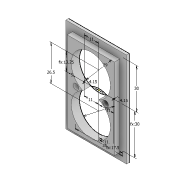
# Autodesk Inventor part: sf11c_lidar_mount
Saved by Autodesk Inventor 2022 (Build 260153000, 153)
## iProperties
Created: 2022-05-19
Part Number: sf11c_lidar_mount
Material: Generic
Document SubType Name: Modeling
Designer: Thomas
Density: 1 g/cm^3
Appearance: Default
Author: Thomas
Autodesk Inventor part; units mm, degrees
ref_plane "YZ Plane" through (0, 0, 0) normal (1, 0, 0) x (0, 1, 0)
ref_plane "XZ Plane" through (0, 0, 0) normal (0, 1, 0) x (-1, 0, 0)
ref_plane "XY Plane" through (0, 0, 0) normal (0, 0, 1) x (1, 0, 0)
sketch "Sketch1" plane through (0, 0, 0) normal (0, 0, 1) x (1, 0, 0)
  circle A0 centre (0, 13.25) radius 14.5
  circle A1 centre (0, -13.25) radius 14.5
  line L0 (0, 13.25) -> (0, -13.25) construction
  circle A2 centre (11, 0) radius 2.075
  circle A3 centre (-11, 0) radius 2.075
  line L1 (-17.5, 30) -> (17.5, 30)
  line L2 (17.5, 30) -> (17.5, -30)
  line L3 (17.5, -30) -> (-17.5, -30)
  line L4 (-17.5, -30) -> (-17.5, 30)
  line L5 (-22.5, 35) -> (22.5, 35)
  line L6 (22.5, 35) -> (22.5, -35)
  line L7 (22.5, -35) -> (-22.5, -35)
  line L8 (-22.5, -35) -> (-22.5, 35)
  point P0 (0, 0)
  point P1 (-5.8896, 0)
  point P2 (5.8896, 0)
  dimension "d0" = 29
  dimension "d1" = 29
  dimension "d2" = 26.5
  dimension "d3" = 13.25
  dimension "d6" = 0
  dimension "d7" = 4.15
  dimension "d8" = 4.15
  dimension "d9" = 11
  dimension "d10" = 11
  dimension "d11" = 11
  dimension "d12" = 11
  dimension "d13" = 35
  dimension "d14" = 17.5
  dimension "d15" = 30
  dimension "d16" = 30
  dimension "d17" = 5
  constraints: 18 end point, 4 centre point, 4 parallel, 2 perpendicular, 1 horizontal, 1 vertical, 3 other
  measures "d0" diameter of A0
  measures "d1" diameter of A1
  measures "d2" distance of L0.start L0.end
  measures "d3" distance of point (0, 0) L0.start
  measures "d6" distance from line of point (0, 0) L0
  measures "d7" diameter of A2
  measures "d8" diameter of A3
  measures "d9" distance of A3.centre point (0, 0)
  measures "d10" distance of A2.centre point (0, 0)
  measures "d11" distance from line of A2.centre L0
  measures "d12" distance from line of A3.centre L0
  measures "d13" distance of L2.end L3.end
  measures "d14" distance from line of point (0, 0) L2
  measures "d15" distance from line of point (0, 0) L1
  measures "d16" distance from line of point (0, 0) L3
  measures "d17" distance between parallel lines of L4 L8
extrude "Extrusion1" add sketch "Sketch1" along normal blind 2 contours L1 L2 L3 L4 | L5 L6 L7 L8
extrude "Extrusion2" add sketch "Sketch1" along normal blind 6 contours L1 L2 L3 L4
equation "\"d3\" = 0.5 * d2"
equation "\"d14\" = 0.5 * d13"
equation "\"d16\" = d15"
body "Solid1"
